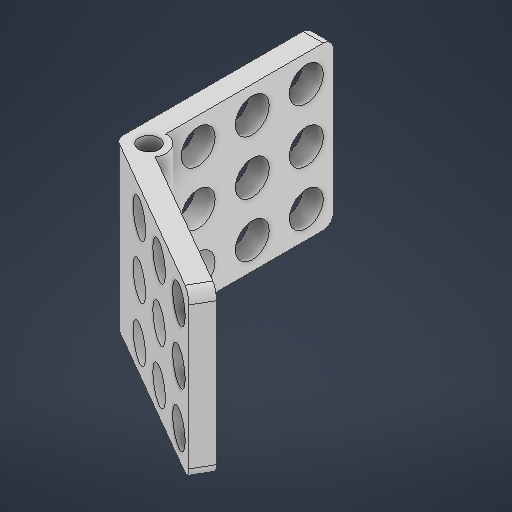
# Autodesk Inventor part: Bracket Bend 3x3
Saved by Autodesk Inventor 2026.1 (Build 301233020, 233B)
## iProperties
Created: 2025-10-18
Part Number: Bracket Bend 3x3
Material: Generic
Document SubType Name: Modeling
Designer: User
Density: 1 g/cm^3
Appearance: Default
Author: User
Autodesk Inventor part; units mm, degrees
ref_plane "YZ Plane" through (0, 0, 0) normal (1, 0, 0) x (0, 1, 0)
ref_plane "XZ Plane" through (0, 0, 0) normal (0, 1, 0) x (-1, 0, 0)
ref_plane "XY Plane" through (0, 0, 0) normal (0, 0, 1) x (1, 0, 0)
sketch "Sketch1" plane through (0, 0, 0) normal (0, 1, 0) x (-1, 0, 0)
  line L0 (0, 0) -> (0, -29)
  line L1 (0, 0) -> (-25.1147, 14.5)
  line L2 (0, 0) -> (29, 0) construction
  line L3 (0, -29) -> (-3, -29)
  line L4 (-3, -29) -> (-3, -4.2321)
  line L5 (-25.1147, 14.5) -> (-26.6147, 11.9019)
  line L6 (-26.6147, 11.9019) -> (-5.1651, -0.4821)
  arc A0 (-5.1651, -0.4821) -> (-3, -4.2321) centre (-3, -1.7321) ccw
  circle A1 centre (-3, -1.7321) radius 1.5
  constraints: 14 end point, 2 centre point, 2 horizontal, 2 point on circle, 1 coincident, 1 equal length, 1 perpendicular, 1 vertical
extrude "Extrusion1" add sketch "Sketch1" along normal blind 24
fillet "Fillet1" radius 1.5 1 edges at (1.5, 24, -29)
fillet "Fillet2" radius 1.5 3 edges at (25.8647, 24, 13.201) (25.8647, 0, 13.201) (1.5, 0, -29)
sketch "Sketch2" plane through (3, 0, -4.2321) normal (1, 0, 0) x (0, 0, -1)
  line L0 (0, 0) -> (23.2679, 0) projected
  circle A0 centre (20.768, 20) radius 2.5
  circle A1 centre (20.7679, 12) radius 2.5
  circle A2 centre (20.7679, 4) radius 2.5
  line L1 (24.7679, 1.5) -> (24.7679, 22.5) projected
  circle A3 centre (4.768, 20) radius 2.5
  circle A4 centre (12.768, 20) radius 2.5
  circle A5 centre (12.768, 12) radius 2.5
  circle A6 centre (12.768, 4) radius 2.5
  circle A7 centre (4.768, 4) radius 2.5
  circle A8 centre (4.768, 12) radius 2.5
  point P0 (-4.2321, 0)
  constraints: 9 centre point
sketch "Sketch3" plane through (5.1651, 0, -0.4821) normal (0.5, 0, -0.866) x (-0.866, 0, -0.5)
  circle A0 centre (-20.7679, 20) radius 2.5
  circle A1 centre (-20.7679, 12) radius 2.5
  circle A2 centre (-20.7679, 4) radius 2.5
  circle A3 centre (-12.7679, 4) radius 2.5
  circle A4 centre (-12.7679, 12) radius 2.5
  circle A5 centre (-12.7679, 20) radius 2.5
  circle A6 centre (-4.7679, 20) radius 2.5
  circle A7 centre (-4.7679, 12) radius 2.5
  circle A8 centre (-4.7679, 4) radius 2.5
  point P0 (4.2321, 0)
  constraints: 9 centre point
extrude "Extrusion2" cut sketch "Sketch3" against normal blind 24 contours A2
extrude "Extrusion3" cut sketch "Sketch3" against normal blind 24 contours A0 | A1 | A3 | A4 | A5 | A6 | A7 | A8
extrude "Extrusion4" cut sketch "Sketch2" against normal blind 24
fillet "Fillet3" radius 1.5 1 edges at (0, 12, 0)
body "Solid1"
